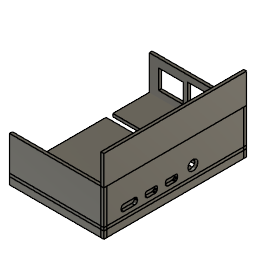
RaspberryPI_Halterung (Autodesk Fusion 360 design; units mm, degrees)
Autodesk Fusion 360 part; units mm, degrees
box "Grundkörper Quader1" add length 96 width 63.5 height 2 placed x (0, -1, 0) y (1, 0, 0) z (0, 0, 1) at (0, 0, 0) makes body 1 in component "RaspberryPI"
box "Grundkörper Quader2" add length 2 width 63.5 height 30 placed x (0, -1, 0) y (1, 0, 0) z (0, 0, 1) at (0, 0, 0) separate body makes body 2 in component "RaspberryPI"
box "Grundkörper Quader3" add length 2 width 63.5 height 30 placed x (0, 1, 0) y (-1, 0, 0) z (0, 0, 1) at (63.5, -96, 0) separate body makes body 3 in component "RaspberryPI"
box "Grundkörper Quader4" add length 96 width 2 height 30 placed x (0, -1, 0) y (1, 0, 0) z (0, 0, 1) at (61.5, 0, 0) separate body makes body 4 in component "RaspberryPI"
box "Grundkörper Quader6" cut length 15 width 13.5 height -2 placed x (0, 0, 1) y (1, 0, 0) z (0, 1, 0) at (44.85, 0, 10.75) bodies 2 in component "RaspberryPI"
box "Grundkörper Quader8" cut length 15 width 14.5 height -2 placed x (0, 0, 1) y (1, 0, 0) z (0, 1, 0) at (25.85, 0, 10.75) bodies 2 in component "RaspberryPI"
box "Grundkörper Quader10" cut length 13 width 16.5 height -2 placed x (0, 0, 1) y (1, 0, 0) z (0, 1, 0) at (6.35, 0, 11.2) bodies 2 in component "RaspberryPI"
box "Grundkörper Quader12" cut length 2 width 4.5 height -61 placed x (0, 0, 1) y (0, 1, 0) z (-1, 0, 0) at (0, -31, 0) bodies 1 in component "RaspberryPI"
box "Grundkörper Quader14" cut length 2 width 4.5 height -61 placed x (0, 0, -1) y (0, -1, 0) z (-1, 0, 0) at (0, -84.5, 2) bodies 1 in component "RaspberryPI"
move_body "Verschieben5" bodies 2 4 3 to x (1, 0, 0) y (0, 1, 0) z (0, 0, 1) at (0, 0, -4.85) in component "RaspberryPI"
cylinder "Grundkörper Zylinder1" cut diameter 6.6 height -2 placed x (0, 0, 1) y (0, 1, 0) z (-1, 0, 0) at (61.5, -36.1, 8.35) bodies 4 1 in component "RaspberryPI"
box "Grundkörper Quader17" add length 4 width 8 height 1 placed x (0, 0, 1) y (0, 1, 0) z (-1, 0, 0) at (61.5, -54.5, 4.75) separate body makes body 5 in component "RaspberryPI"
fillet "Abrundung1" radius 0.87 2 edges at (61, -54.5, 8.75) (61, -46.5, 8.75) on bodies 5 in component "RaspberryPI"
box "Grundkörper Quader18" add length 1 width 2 height 1 placed x (0, 0, -1) y (0, -1, 0) z (-1, 0, 0) at (61.5, -46.5, 4.75) separate body makes body 6 in component "RaspberryPI"
move_body "Verschieben2" bodies 6 to x (1, 0, 0) y (0, 0.707107, 0.707107) z (0, -0.707107, 0.707107) at (0, -10.1294, 35.5344) in component "RaspberryPI"
copy_body "Körper kopieren/einfügen2" bodies 6 makes body 7 in component "RaspberryPI"
move_body "Verschieben3" bodies 7 to x (1, 0, 0) y (0, 0, 1) z (0, -1, 0) at (0, -49.3914, 51.6743) in component "RaspberryPI"
combine "Kombinieren1" operation cut target body 5 tool bodies 6 7 in component "RaspberryPI"
fillet "Abrundung2" radius 0.9 4 edges at (61, -54.5, 5.8157) (61, -53.4343, 4.75) (61, -47.6314, 4.75) (61, -46.5, 5.8814) on bodies 5 in component "RaspberryPI"
copy_body "Körper kopieren/einfügen3" bodies 5 makes body 8 in component "RaspberryPI"
move_body "Verschieben4" bodies 8 to x (1, 0, 0) y (0, 1, 0) z (0, 0, 1) at (0, -13.5, 0) in component "RaspberryPI"
extrude "Extrusion1" cut 2 faces at (60.5, -49.6681, 7.4167) (60.5, -63.1681, 7.4167) along direction (1, 0, 0) blind 3 on bodies 5 8 bodies 4 5 8 in component "RaspberryPI"
delete_body "Körper entfernen1" bodies 5 in component "RaspberryPI"
delete_body "Körper entfernen2" bodies 8 in component "RaspberryPI"
box "Grundkörper Quader20" add length 4.3 width 11 height 1 placed x (0, 0, 1) y (0, 1, 0) z (-1, 0, 0) at (61.5, -84.4, 4.75) separate body makes body 9 in component "RaspberryPI"
fillet "Abrundung3" radius 1.84 4 edges at (61, -73.4, 9.05) (61, -73.4, 4.75) (61, -84.4, 9.05) (61, -84.4, 4.75) on bodies 9 in component "RaspberryPI"
extrude "Extrusion2" cut 1 faces at (60.5, -77.68, 6.1833) along direction (1, 0, 0) blind 3 on bodies 9 bodies 4 9 in component "RaspberryPI"
delete_body "Körper entfernen3" bodies 9 in component "RaspberryPI"
extrude "Extrusion3" add 1 faces at (62.8333, -32, 25.15) along direction (0, 0, 1) blind 20 separate body on bodies 4 makes body 10 in component "RaspberryPI"
sketch "Skizze1" plane through (0, -96, 0) normal (0, -1, 0) x (1, 0, 0)
  line L0 (61.5, 25.15) -> (63.5, 25.15)
  line L1 (63.5, 25.15) -> (63.5, 45.15)
  line L2 (63.5, 45.15) -> (61.5, 45.15)
  line L3 (61.5, 45.15) -> (61.5, 25.15)
  line L4 (62.5, 45.15) -> (60.5, 45.15)
  line L5 (60.5, 45.15) -> (62.5, 42.5)
  line L6 (62.5, 42.5) -> (64.5, 45.15)
  line L7 (64.5, 45.15) -> (62.5, 45.15)
  dimension "d115" = 3.32
  constraint midpoint L2 L4.start
  constraint perpendicular L3 L4
  constraint parallel L4 L7
  measures "d115" distance of L5.end L6.end
extrude "Extrusion4" [suppressed] in component "RaspberryPI"
component "RaspberryPI" placed x (1, 0, 0) y (0, 1, 0) z (0, 0, 1) at (0, 0, 0)
named bodies: "Unterteil", "Wand_Vorne", "Wand_Hinten", "Wand_Rechts", "Wand_Clipper"
